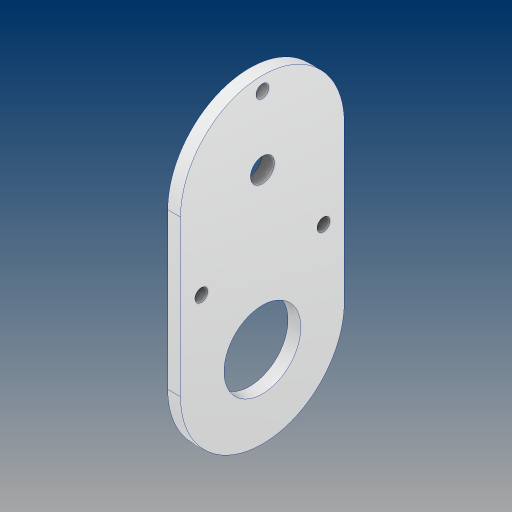
# Autodesk Inventor part: Intake Pulley Cover 1
Saved by Autodesk Inventor 2024.3 (Build 283343000, 343)
## iProperties
Created: 2024-08-03
Part Number: Intake Pulley Cover 1
Material: Aluminum 6061
Document SubType Name: Modeling
Designer: Kenji
Density: 2.7 g/cm^3
Appearance: Aluminum - Flat
Author: Kenji
Autodesk Inventor part; units mm, degrees
ref_plane "YZ Plane" through (0, 0, 0) normal (1, 0, 0) x (0, 1, 0)
ref_plane "XZ Plane" through (0, 0, 0) normal (0, 1, 0) x (-1, 0, 0)
ref_plane "XY Plane" through (0, 0, 0) normal (0, 0, 1) x (1, 0, 0)
sketch "Sketch1" plane through (0, 0, 0) normal (1, 0, 0) x (0, 1, 0)
  circle A0 centre (0, 0) radius 30.48 construction
  circle A1 centre (57.9374, 0) radius 30.48 construction
  line L0 (57.9374, -30.48) -> (0, -30.48)
  line L1 (57.9374, 30.48) -> (0, 30.48)
  circle A2 centre (28.9687, 22.7434) radius 3.81 construction
  circle A3 centre (28.9687, -22.7434) radius 3.81 construction
  line L2 (31.9655, -20.3907) -> (33.9633, -18.8221) construction
  line L3 (25.9719, -20.3907) -> (23.9741, -18.8221) construction
  line L4 (31.9655, 20.3907) -> (33.9633, 18.8221) construction
  line L5 (25.9719, 20.3907) -> (23.9741, 18.8221) construction
  circle A4 centre (57.9374, 0) radius 25.4 construction
  circle A5 centre (57.9374, 0) radius 4.445
  circle A6 centre (83.3374, 0) radius 2.3876
  circle A7 centre (28.9687, 22.7434) radius 2.3876
  circle A8 centre (28.9687, -22.7434) radius 2.3876
  arc A9 (0, 30.48) -> (0, -30.48) centre (0, 0) ccw
  arc A10 (57.9374, -30.48) -> (57.9374, 30.48) centre (57.9374, 0) ccw
  circle A11 centre (0, 0) radius 14.2875
  dimension "d7" = 50.8
  dimension "d0" = 60.96
  dimension "d1" = 60.96
  dimension "d2" = 57.9374
  dimension "d3" = 7.62
  dimension "d4" = 7.62
  dimension "d5" = 2.54
  dimension "d6" = 2.54
  dimension "d8" = 8.89
  dimension "d9" = 4.7752
  dimension "d13" = 4.7752
  dimension "d14" = 4.7752
  dimension "d15" = 28.575
  constraints: 16 point on circle, 12 end point, 11 centre point, 8 point on line, 6 coincident, 6 tangent, 3 horizontal alignment, 2 equal length, 1 concentric, 2 other
  measures "d0" diameter of A0
  measures "d1" diameter of A1
  measures "d2" distance of point (0, 0) A1.centre
  measures "d3" diameter of A2
  measures "d4" diameter of A3
  measures "d5" distance of L4.start L4.end
  measures "d6" distance of L2.start L2.end
  measures "d8" diameter of A5
  measures "d9" diameter of A6
  measures "d13" diameter of A7
  measures "d14" diameter of A8
  measures "d15" diameter of A11
extrude "Extrusion1" add sketch "Sketch1" along normal blind 4.7625
body "Solid1"
